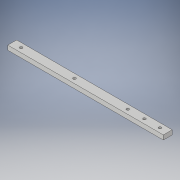
# Autodesk Inventor part: batang_horn_normal
Saved by Autodesk Inventor 2019 (Build 230136000, 136)
## iProperties
Created: 2020-07-19
Part Number: batang_horn_normal
Material: Generic
Document SubType Name: Modeling
Designer: Agus Prayudi
Density: 1 g/cm^3
Appearance: Default
Author: Agus Prayudi
Autodesk Inventor part; units mm, degrees
ref_plane "YZ Plane" through (0, 0, 0) normal (1, 0, 0) x (0, 1, 0)
ref_plane "XZ Plane" through (0, 0, 0) normal (0, 1, 0) x (-1, 0, 0)
ref_plane "XY Plane" through (0, 0, 0) normal (0, 0, 1) x (1, 0, 0)
sketch "Sketch1" plane through (0, 0, 0) normal (0, 1, 0) x (-1, 0, 0)
  line L0 (70, 5) -> (-70, 5)
  line L1 (-70, -5) -> (70, -5)
  line L2 (70, -5) -> (70, 5)
  line L3 (-70, -5) -> (-105, -5)
  line L4 (-105, -5) -> (-105, 5)
  line L5 (-105, 5) -> (-70, 5)
  circle A0 centre (-78.75, 0) radius 1.5
  circle A1 centre (-96.25, 0) radius 1.5
  circle A2 centre (0, 0) radius 1.5
  circle A3 centre (60, 0) radius 1.5
  circle A4 centre (-60, 0) radius 1.5
  constraints: 12 end point, 5 centre point, 2 perpendicular, 1 coincident, 1 horizontal, 1 parallel, 1 point on line
extrude "Extrusion1" add sketch "Sketch1" along normal blind 5
body "Solid1"
